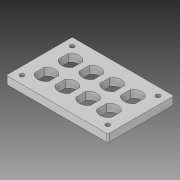
# Autodesk Inventor part: 4_OM_VialPlate_0.25mmReduce
Saved by Autodesk Inventor 2019 (Build 230136000, 136)
## iProperties
Created: 2020-06-22
Part Number: 4_OM_VialPlate_0.25mmReduce
Material: Generic
Document SubType Name: Modeling
Designer: devon
Density: 1 g/cm^3
Appearance: Default
Author: devon
Autodesk Inventor part; units mm, degrees
ref_plane "YZ Plane" through (0, 0, 0) normal (1, 0, 0) x (0, 1, 0)
ref_plane "XZ Plane" through (0, 0, 0) normal (0, 1, 0) x (-1, 0, 0)
ref_plane "XY Plane" through (0, 0, 0) normal (0, 0, 1) x (1, 0, 0)
sketch "Sketch1" plane through (0, 0, 0) normal (0, 1, 0) x (-1, 0, 0)
  line L0 (80, 52) -> (-80, 52)
  line L1 (-80, 52) -> (-80, -52)
  line L2 (-80, -52) -> (80, -52)
  line L3 (80, -52) -> (80, 52)
  line L4 (80, 52) -> (-80, -52) construction
  line L5 (-80, 52) -> (80, -52) construction
  point P0 (0, 0)
  dimension "d0" = 160
  dimension "d1" = 104
  constraints: 12 end point, 2 midpoint, 2 parallel, 1 horizontal, 1 perpendicular
  measures "d0" distance of L1.end L2.end
  measures "d1" distance of L2.end L0.start
extrude "Extrusion1" add sketch "Sketch1" along normal blind 12
sketch "Sketch2" plane through (0, 12, 0) normal (0, 1, 0) x (1, 0, 0)
  line L0 (-80, 52) -> (-80, -52) projected
  line L1 (80, 52) -> (-80, 52) projected
  line L2 (-38.125, 26.75) -> (-38.125, 11)
  line L3 (-60.875, 11) -> (-60.875, 26.75)
  arc A0 (-38.125, 26.75) -> (-60.875, 26.75) centre (-49.5, 18.875) ccw
  arc A1 (-60.875, 11) -> (-38.125, 11) centre (-49.5, 18.875) ccw
  point P0 (0, 0)
  dimension "d39" = 22.75
  dimension "d40" = 15.75
  dimension "d41" = 19.125
  dimension "d42" = 7.875
  dimension "d43" = 33.125
  constraints: 4 end point, 4 point on circle, 2 centre point, 1 coincident, 1 parallel
  measures "d39" distance of L3.end L2.start
  measures "d40" distance of L3.start L3.end
  measures "d41" distance between parallel lines of L0 L3
  measures "d42" vertical distance of L2.start A0.centre
  measures "d43" distance from line of L1 A0.centre
extrude "Extrusion2" cut sketch "Sketch2" against normal up to next
pattern_linear "Rectangular Pattern1" count 4 spacing -32.75 along (-1, 0, 0) count 2 spacing 37.75 along (0, 0, 1) of "Extrusion2"
sketch "Sketch4" plane through (0, 12, 0) normal (0, 1, 0) x (1, 0, 0)
  line L0 (-80, 52) -> (-80, -52) projected
  line L1 (80, 52) -> (-80, 52) projected
  line L2 (80, -52) -> (80, 52) projected
  line L3 (-80, -52) -> (80, -52) projected
  point P0 (0, 0)
  point P1 (-67.5, 39.5)
  point P2 (67.5, 39.5)
  point P3 (67.5, -39.5)
  point P4 (-67.5, -39.5)
  dimension "d24" = 12.5
  dimension "d25" = 12.5
  dimension "d26" = 12.5
  dimension "d27" = 12.5
  dimension "d28" = 12.5
  dimension "d29" = 12.5
  dimension "d30" = 12.5
  dimension "d31" = 12.5
  measures "d24" distance from line of L0 point (-67.5, 39.5)
  measures "d25" distance from line of L1 point (-67.5, 39.5)
  measures "d26" distance from line of L2 point (67.5, 39.5)
  measures "d27" distance from line of L1 point (67.5, 39.5)
  measures "d28" distance from line of L2 point (67.5, -39.5)
  measures "d29" distance from line of L3 point (67.5, -39.5)
  measures "d30" distance from line of L3 point (-67.5, -39.5)
  measures "d31" distance from line of L0 point (-67.5, -39.5)
hole "Hole1" at (-67.5, 12, -39.5) at (67.5, 12, -39.5) at (67.5, 12, 39.5) at (-67.5, 12, 39.5) direction (0, -1, 0) diameter 6.756 depth 25.4 clearance for "Socket Head Cap Screw" size "1/4" standard "Ansi Unified Screw Threads"
fillet "Fillet1" radius 2 4 edges at (-80, 6, 52) (80, 6, 52) (80, 6, -52) (-80, 6, -52)
body "Solid1"
